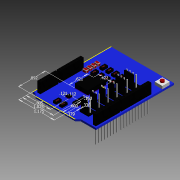
# Autodesk Inventor part: GBS-20132-EL2
Saved by Autodesk Inventor 2013 (Build 170138000, 138)
## iProperties
Created: 2013-09-06
Part Number: GBS-20132-EL2
Material: Generic
Document SubType Name: Modeling
Designer: HP_Administrator
Density: 1 g/cm^3
GlobalPropertyList: <PropertyList/>
Author: HP_Administrator
Autodesk Inventor part; units mm, degrees
(part 1 of 2)
ref_plane "YZ Plane" through (0, 0, 0) normal (1, 0, 0) x (0, 1, 0)
ref_plane "XZ Plane" through (0, 0, 0) normal (0, 1, 0) x (-1, 0, 0)
ref_plane "XY Plane" through (0, 0, 0) normal (0, 0, 1) x (1, 0, 0)
sketch "Sketch1" plane through (0, 0, 0) normal (0, 1, 0) x (-1, 0, 0)
  line L0 (26.67, -33.02) -> (-26.67, -33.02)
  line L1 (-26.67, -33.02) -> (-26.67, 33.02)
  line L2 (26.67, -33.02) -> (26.67, 33.02)
  line L3 (26.67, 33.02) -> (24.638, 33.02)
  line L4 (-26.67, 33.02) -> (-13.97, 33.02)
  line L5 (22.0345, 35.306) -> (-11.3665, 35.306)
  line L6 (24.638, 33.02) -> (22.0345, 35.306)
  line L7 (-11.3665, 35.306) -> (-13.97, 33.02)
  line L8 (26.67, -33.02) -> (-26.67, 33.02) construction
  line L9 (26.67, 33.02) -> (-26.67, -33.02) construction
  point P0 (0, 0)
  point P1 (0, 0)
  point P2 (0, 0)
  dimension "d0" = 53.34
  dimension "d1" = 66.04
  dimension "d2" = 66.04
  dimension "d3" = 2.032
  dimension "d4" = 12.7
  dimension "d5" = 2.286
  dimension "d6" = 33.401
  constraints: 20 end point, 2 midpoint, 2 parallel, 2 perpendicular, 1 coincident, 1 collinear, 1 equal length, 1 horizontal
  measures "d0" distance of L0.start L0.end
  measures "d1" distance of L0.end L1.end
  measures "d2" distance of L0.start L2.end
  measures "d3" distance of L2.end L3.end
  measures "d4" distance of L1.end L4.end
  measures "d5" distance between parallel lines of L4 L5
  measures "d6" distance of L5.start L5.end
extrude "PCB BD" add sketch "Sketch1" along normal blind 1.524
sketch "Sketch2" plane through (0, 1.524, 0) normal (0, 1, 0) x (1, 0, 0)
  line L0 (26.67, 33.02) -> (-26.67, 33.02) projected
  line L1 (-22.0345, -35.306) -> (11.3665, -35.306) projected
  line L2 (26.67, -33.02) -> (26.67, 33.02) projected
  line L3 (-4.8895, -32.766) -> (-2.2225, -32.766)
  line L4 (-2.2225, -32.766) -> (-2.2225, -28.1305)
  line L5 (-2.2225, -28.1305) -> (-4.8895, -28.1305)
  line L6 (-4.8895, -28.1305) -> (-4.8895, -32.766)
  line L7 (-7.1755, -32.766) -> (-9.8425, -32.766)
  line L8 (-9.8425, -32.766) -> (-9.8425, -28.1305)
  line L9 (-9.8425, -28.1305) -> (-7.1755, -28.1305)
  line L10 (-7.1755, -28.1305) -> (-7.1755, -32.766)
  line L11 (-0.127, 16.2179) -> (2.54, 16.2179)
  line L12 (2.54, 16.2179) -> (2.54, 11.5824)
  line L13 (2.54, 11.5824) -> (-0.127, 11.5824)
  line L14 (-0.127, 11.5824) -> (-0.127, 16.2179)
  line L15 (-2.413, 11.5824) -> (-5.08, 11.5824)
  line L16 (-5.08, 11.5824) -> (-5.08, 16.2179)
  line L17 (-5.08, 16.2179) -> (-2.413, 16.2179)
  line L18 (-2.413, 16.2179) -> (-2.413, 11.5824)
  line L19 (-7.366, 11.5824) -> (-10.033, 11.5824)
  line L20 (-10.033, 11.5824) -> (-10.033, 16.2179)
  line L21 (-10.033, 16.2179) -> (-7.366, 16.2179)
  line L22 (-7.366, 16.2179) -> (-7.366, 11.5824)
  line L23 (-12.319, 11.5824) -> (-14.986, 11.5824)
  line L24 (-14.986, 11.5824) -> (-14.986, 16.2179)
  line L25 (-14.986, 16.2179) -> (-12.319, 16.2179)
  line L26 (-12.319, 16.2179) -> (-12.319, 11.5824)
  line L27 (-14.986, 8.5344) -> (-12.319, 8.5344)
  line L28 (-12.319, 8.5344) -> (-12.319, 3.8989)
  line L29 (-12.319, 3.8989) -> (-14.986, 3.8989)
  line L30 (-14.986, 3.8989) -> (-14.986, 8.5344)
  line L31 (-10.033, 8.5344) -> (-7.366, 8.5344)
  line L32 (-7.366, 8.5344) -> (-7.366, 3.8989)
  line L33 (-7.366, 3.8989) -> (-10.033, 3.8989)
  line L34 (-10.033, 3.8989) -> (-10.033, 8.5344)
  line L35 (-5.08, 8.5344) -> (-2.413, 8.5344)
  line L36 (-2.413, 8.5344) -> (-2.413, 3.8989)
  line L37 (-2.413, 3.8989) -> (-5.08, 3.8989)
  line L38 (-5.08, 3.8989) -> (-5.08, 8.5344)
  line L39 (-0.127, 8.5344) -> (2.54, 8.5344)
  line L40 (2.54, 8.5344) -> (2.54, 3.8989)
  line L41 (2.54, 3.8989) -> (-0.127, 3.8989)
  line L42 (-0.127, 3.8989) -> (-0.127, 8.5344)
  point P0 (0, 0)
  dimension "d9" = 2.54
  dimension "d10" = 4.6355
  dimension "d11" = 2.667
  dimension "d13" = 28.8925
  dimension "d14" = 2.286
  dimension "d15" = 16.8021
  dimension "d16" = 24.13
  dimension "d17" = 2.286
  dimension "d18" = 2.286
  dimension "d19" = 2.286
  dimension "d20" = 3.048
  constraints: 80 end point, 20 parallel, 18 equal length, 11 collinear, 10 horizontal, 10 perpendicular
  measures "d9" distance between parallel lines of L1 L3
  measures "d10" distance of L3.end L4.end
  measures "d11" distance of L4.end L5.end
  measures "d13" distance between parallel lines of L2 L4
  measures "d14" distance between parallel lines of L10 L6
  measures "d15" distance between parallel lines of L0 L11
  measures "d16" distance between parallel lines of L2 L12
  measures "d17" distance between parallel lines of L18 L14
  measures "d18" distance between parallel lines of L22 L16
  measures "d19" distance between parallel lines of L26 L20
  measures "d20" distance between parallel lines of L27 L23
extrude "SK14 GP" add sketch "Sketch2" along normal blind 1.778
sketch "Sketch3" plane through (0, 3.302, 0) normal (0, 1, 0) x (1, 0, 0)
  line L0 (-2.2225, -32.766) -> (-2.2225, -28.1305) projected
  line L1 (-14.986, 11.5824) -> (-12.319, 11.5824) projected
  line L2 (-12.319, 11.5824) -> (-12.319, 16.2179) projected
  line L3 (-12.319, 16.2179) -> (-14.986, 16.2179) projected
  line L4 (-14.986, 16.2179) -> (-14.986, 11.5824) projected
  line L5 (-10.033, 11.5824) -> (-7.366, 11.5824) projected
  line L6 (-7.366, 11.5824) -> (-7.366, 16.2179) projected
  line L7 (-7.366, 16.2179) -> (-10.033, 16.2179) projected
  line L8 (-10.033, 16.2179) -> (-10.033, 11.5824) projected
  line L9 (-5.08, 11.5824) -> (-2.413, 11.5824) projected
  line L10 (-2.413, 11.5824) -> (-2.413, 16.2179) projected
  line L11 (-2.413, 16.2179) -> (-5.08, 16.2179) projected
  line L12 (-5.08, 16.2179) -> (-5.08, 11.5824) projected
  line L13 (2.54, 16.2179) -> (-0.127, 16.2179) projected
  line L14 (-0.127, 16.2179) -> (-0.127, 11.5824) projected
  line L15 (-0.127, 11.5824) -> (2.54, 11.5824) projected
  line L16 (2.54, 11.5824) -> (2.54, 16.2179) projected
  line L17 (2.54, 8.5344) -> (-0.127, 8.5344) projected
  line L18 (-0.127, 8.5344) -> (-0.127, 3.8989) projected
  line L19 (-0.127, 3.8989) -> (2.54, 3.8989) projected
  line L20 (2.54, 3.8989) -> (2.54, 8.5344) projected
  line L21 (-2.413, 8.5344) -> (-5.08, 8.5344) projected
  line L22 (-5.08, 8.5344) -> (-5.08, 3.8989) projected
  line L23 (-5.08, 3.8989) -> (-2.413, 3.8989) projected
  line L24 (-2.413, 3.8989) -> (-2.413, 8.5344) projected
  line L25 (-7.366, 8.5344) -> (-10.033, 8.5344) projected
  line L26 (-10.033, 8.5344) -> (-10.033, 3.8989) projected
  line L27 (-10.033, 3.8989) -> (-7.366, 3.8989) projected
  line L28 (-7.366, 3.8989) -> (-7.366, 8.5344) projected
  line L29 (-12.319, 8.5344) -> (-14.986, 8.5344) projected
  line L30 (-14.986, 8.5344) -> (-14.986, 3.8989) projected
  line L31 (-14.986, 3.8989) -> (-12.319, 3.8989) projected
  line L32 (-12.319, 3.8989) -> (-12.319, 8.5344) projected
  line L33 (-9.8425, -32.766) -> (-7.1755, -32.766) projected
  line L34 (-9.8425, -32.766) -> (-7.1755, -32.766) projected
  line L35 (-7.1755, -32.766) -> (-7.1755, -28.1305) projected
  line L36 (-7.1755, -28.1305) -> (-9.8425, -28.1305) projected
  line L37 (-9.8425, -28.1305) -> (-9.8425, -32.766) projected
  line L38 (-7.6327, -29.7815) -> (-7.6327, -32.766) construction
  line L39 (-7.6327, -32.766) -> (-9.8425, -32.766) construction
  line L40 (-9.8425, -32.766) -> (-9.8425, -29.7815) construction
  line L41 (-9.8425, -29.7815) -> (-7.6327, -29.7815) construction
  line L42 (-2.6797, -29.7815) -> (-2.6797, -32.766) construction
  line L43 (-2.6797, -32.766) -> (-4.8895, -32.766) construction
  line L44 (-4.8895, -32.766) -> (-4.8895, -29.7815) construction
  line L45 (-4.8895, -29.7815) -> (-2.6797, -29.7815) construction
  line L46 (2.0828, 14.5669) -> (2.0828, 11.5824) construction
  line L47 (2.0828, 11.5824) -> (-0.127, 11.5824) construction
  line L48 (-0.127, 11.5824) -> (-0.127, 14.5669) construction
  line L49 (-0.127, 14.5669) -> (2.0828, 14.5669) construction
  line L50 (-12.9587, 6.8834) -> (-12.9587, 3.8989) construction
  line L51 (-12.9587, 3.8989) -> (-14.986, 3.8989) construction
  line L52 (-14.986, 3.8989) -> (-14.986, 6.8834) construction
  line L53 (-14.986, 6.8834) -> (-12.9587, 6.8834) construction
  line L54 (-7.8232, 6.8834) -> (-7.8232, 3.8989) construction
  line L55 (-7.8232, 3.8989) -> (-10.033, 3.8989) construction
  line L56 (-10.033, 3.8989) -> (-10.033, 6.8834) construction
  line L57 (-10.033, 6.8834) -> (-7.8232, 6.8834) construction
  line L58 (-12.9587, 14.5669) -> (-12.9587, 11.5824) construction
  line L59 (-12.9587, 11.5824) -> (-14.986, 11.5824) construction
  line L60 (-14.986, 11.5824) -> (-14.986, 14.5669) construction
  line L61 (-14.986, 14.5669) -> (-12.9587, 14.5669) construction
  line L62 (-7.8232, 14.5669) -> (-7.8232, 11.5824) construction
  line L63 (-7.8232, 11.5824) -> (-10.033, 11.5824) construction
  line L64 (-10.033, 11.5824) -> (-10.033, 14.5669) construction
  line L65 (-10.033, 14.5669) -> (-7.8232, 14.5669) construction
  line L66 (-2.8702, 14.5669) -> (-2.8702, 11.5824) construction
  line L67 (-2.8702, 11.5824) -> (-5.08, 11.5824) construction
  line L68 (-5.08, 11.5824) -> (-5.08, 14.5669) construction
  line L69 (-5.08, 14.5669) -> (-2.8702, 14.5669) construction
  line L70 (-5.08, 6.8834) -> (-2.8702, 6.8834) construction
  line L71 (-2.8702, 6.8834) -> (-2.8702, 3.8989) construction
  line L72 (-2.8702, 3.8989) -> (-5.08, 3.8989) construction
  line L73 (-5.08, 3.8989) -> (-5.08, 6.8834) construction
  line L74 (-0.127, 6.8834) -> (2.0828, 6.8834) construction
  line L75 (2.0828, 6.8834) -> (2.0828, 3.8989) construction
  line L76 (2.0828, 3.8989) -> (-0.127, 3.8989) construction
  line L77 (-0.127, 3.8989) -> (-0.127, 6.8834) construction
  spline S0 degree 2 poles (-8.4482, -30.0808) (-8.4482, -29.9953) (-8.4124, -29.8753) (-8.3869, -29.8223) knots 0 0 0 1 2 2 2
  line L78 (-8.3869, -29.8223) -> (-8.2555, -29.8223)
  line L79 (-8.2555, -29.8223) -> (-8.2555, -29.83)
  spline S1 degree 2 poles (-8.2555, -29.83) (-8.304, -29.8817) (-8.3576, -30.0125) (-8.3576, -30.0731) knots 0 0 0 1 2 2 2
  spline S2 degree 2 poles (-8.3576, -30.0731) (-8.3576, -30.1599) (-8.2855, -30.2486) (-8.2261, -30.2486) knots 0 0 0 1 2 2 2
  spline S3 degree 2 poles (-8.2261, -30.2486) (-8.1789, -30.2486) (-8.1202, -30.202) (-8.1055, -30.1516) knots 0 0 0 1 2 2 2
  spline S4 degree 2 poles (-8.1055, -30.1516) (-8.0953, -30.1152) (-8.0813, -30.0546) (-8.0698, -30.0093) knots 0 0 0 1 2 2 2
  spline S5 degree 2 poles (-8.0698, -30.0093) (-8.0589, -29.9685) (-8.0264, -29.904) (-8.0002, -29.8791) knots 0 0 0 1 2 2 2
  spline S6 degree 2 poles (-8.0002, -29.8791) (-7.9741, -29.8549) (-7.9039, -29.8281) (-7.8579, -29.8281) knots 0 0 0 1 2 2 2
  spline S7 degree 2 poles (-7.8579, -29.8281) (-7.7622, -29.8281) (-7.6327, -29.9774) (-7.6327, -30.0929) knots 0 0 0 1 2 2 2
  spline S8 degree 2 poles (-7.6327, -30.0929) (-7.6327, -30.1592) (-7.6589, -30.2767) (-7.6837, -30.3271) knots 0 0 0 1 2 2 2
  line L80 (-7.6837, -30.3271) -> (-7.8088, -30.3271)
  line L81 (-7.8088, -30.3271) -> (-7.8088, -30.3194)
  spline S9 degree 2 poles (-7.8088, -30.3194) (-7.7744, -30.2818) (-7.7233, -30.1644) (-7.7233, -30.0999) knots 0 0 0 1 2 2 2
  spline S10 degree 2 poles (-7.7233, -30.0999) (-7.7233, -30.0272) (-7.7916, -29.9372) (-7.8471, -29.9372) knots 0 0 0 1 2 2 2
  spline S11 degree 2 poles (-7.8471, -29.9372) (-7.8969, -29.9372) (-7.9562, -29.9902) (-7.9696, -30.0399) knots 0 0 0 1 2 2 2
  spline S12 degree 2 poles (-7.9696, -30.0399) (-7.9785, -30.0731) (-8.0015, -30.1695) (-8.0111, -30.2014) knots 0 0 0 1 2 2 2
  spline S13 degree 2 poles (-8.0111, -30.2014) (-8.036, -30.2824) (-8.1362, -30.3577) (-8.2095, -30.3577) knots 0 0 0 1 2 2 2
  spline S14 degree 2 poles (-8.2095, -30.3577) (-8.2561, -30.3577) (-8.3454, -30.32) (-8.3767, -30.2862) knots 0 0 0 1 2 2 2
  spline S15 degree 2 poles (-8.3767, -30.2862) (-8.4112, -30.2486) (-8.4482, -30.1529) (-8.4482, -30.0808) knots 0 0 0 1 2 2 2
  line L82 (-8.4341, -31.0385) -> (-8.4341, -30.9026)
  line L83 (-8.4341, -30.9026) -> (-8.0679, -30.6148)
  line L84 (-8.0679, -30.6148) -> (-8.1196, -30.5689)
  line L85 (-8.1196, -30.5689) -> (-8.4341, -30.5689)
  line L86 (-8.4341, -30.5689) -> (-8.4341, -30.4643)
  line L87 (-8.4341, -30.4643) -> (-7.6467, -30.4643)
  line L88 (-7.6467, -30.4643) -> (-7.6467, -30.5689)
  line L89 (-7.6467, -30.5689) -> (-8.0085, -30.5689)
  line L90 (-8.0085, -30.5689) -> (-7.6467, -30.8918)
  line L91 (-7.6467, -30.8918) -> (-7.6467, -31.0194)
  line L92 (-7.6467, -31.0194) -> (-7.9983, -30.6933)
  line L93 (-7.9983, -30.6933) -> (-8.4341, -31.0385)
  line L94 (-8.4341, -31.5248) -> (-8.4341, -31.1406)
  line L95 (-8.4341, -31.1406) -> (-8.3537, -31.1406)
  line L96 (-8.3537, -31.1406) -> (-8.3537, -31.2836)
  line L97 (-8.3537, -31.2836) -> (-7.826, -31.2836)
  line L98 (-7.826, -31.2836) -> (-7.826, -31.1406)
  line L99 (-7.826, -31.1406) -> (-7.7539, -31.1406)
  spline S16 degree 2 poles (-7.7539, -31.1406) (-7.7539, -31.2217) (-7.708, -31.2982) (-7.6442, -31.3033) knots 0 0 0 1 2 2 2
  line L100 (-7.6442, -31.3033) -> (-7.6442, -31.385)
  line L101 (-7.6442, -31.385) -> (-8.3537, -31.385)
  line L102 (-8.3537, -31.385) -> (-8.3537, -31.5248)
  line L103 (-8.3537, -31.5248) -> (-8.4341, -31.5248)
  line L104 (-8.1636, -32.1762) -> (-8.1636, -32.0824)
  line L105 (-8.1636, -32.0824) -> (-8.4341, -32.0824)
  line L106 (-8.4341, -32.0824) -> (-8.4341, -31.981)
  line L107 (-8.4341, -31.981) -> (-8.1636, -31.981)
  line L108 (-8.1636, -31.981) -> (-8.1636, -31.6332)
  line L109 (-8.1636, -31.6332) -> (-8.0526, -31.6332)
  line L110 (-8.0526, -31.6332) -> (-7.6467, -31.9855)
  line L111 (-7.6467, -31.9855) -> (-7.6467, -32.0824)
  line L112 (-7.6467, -32.0824) -> (-8.0787, -32.0824)
  line L113 (-8.0787, -32.0824) -> (-8.0787, -32.1762)
  line L114 (-8.0787, -32.1762) -> (-8.1636, -32.1762)
  line L115 (-8.0787, -31.981) -> (-7.7712, -31.981)
  line L116 (-7.7712, -31.981) -> (-8.0787, -31.7162)
  line L117 (-8.0787, -31.7162) -> (-8.0787, -31.981)
  spline S17 degree 2 poles (-3.4952, -30.0808) (-3.4952, -29.9953) (-3.4594, -29.8753) (-3.4339, -29.8223) knots 0 0 0 1 2 2 2
  line L118 (-3.4339, -29.8223) -> (-3.3025, -29.8223)
  line L119 (-3.3025, -29.8223) -> (-3.3025, -29.83)
  spline S18 degree 2 poles (-3.3025, -29.83) (-3.351, -29.8817) (-3.4046, -30.0125) (-3.4046, -30.0731) knots 0 0 0 1 2 2 2
  spline S19 degree 2 poles (-3.4046, -30.0731) (-3.4046, -30.1599) (-3.3325, -30.2486) (-3.2731, -30.2486) knots 0 0 0 1 2 2 2
  spline S20 degree 2 poles (-3.2731, -30.2486) (-3.2259, -30.2486) (-3.1672, -30.202) (-3.1525, -30.1516) knots 0 0 0 1 2 2 2
  spline S21 degree 2 poles (-3.1525, -30.1516) (-3.1423, -30.1152) (-3.1283, -30.0546) (-3.1168, -30.0093) knots 0 0 0 1 2 2 2
  spline S22 degree 2 poles (-3.1168, -30.0093) (-3.1059, -29.9685) (-3.0734, -29.904) (-3.0472, -29.8791) knots 0 0 0 1 2 2 2
  spline S23 degree 2 poles (-3.0472, -29.8791) (-3.0211, -29.8549) (-2.9509, -29.8281) (-2.9049, -29.8281) knots 0 0 0 1 2 2 2
  spline S24 degree 2 poles (-2.9049, -29.8281) (-2.8092, -29.8281) (-2.6797, -29.9774) (-2.6797, -30.0929) knots 0 0 0 1 2 2 2
  spline S25 degree 2 poles (-2.6797, -30.0929) (-2.6797, -30.1592) (-2.7059, -30.2767) (-2.7307, -30.3271) knots 0 0 0 1 2 2 2
  line L120 (-2.7307, -30.3271) -> (-2.8558, -30.3271)
  line L121 (-2.8558, -30.3271) -> (-2.8558, -30.3194)
  spline S26 degree 2 poles (-2.8558, -30.3194) (-2.8214, -30.2818) (-2.7703, -30.1644) (-2.7703, -30.0999) knots 0 0 0 1 2 2 2
  spline S27 degree 2 poles (-2.7703, -30.0999) (-2.7703, -30.0272) (-2.8386, -29.9372) (-2.8941, -29.9372) knots 0 0 0 1 2 2 2
  spline S28 degree 2 poles (-2.8941, -29.9372) (-2.9439, -29.9372) (-3.0032, -29.9902) (-3.0166, -30.0399) knots 0 0 0 1 2 2 2
  spline S29 degree 2 poles (-3.0166, -30.0399) (-3.0255, -30.0731) (-3.0485, -30.1695) (-3.0581, -30.2014) knots 0 0 0 1 2 2 2
  spline S30 degree 2 poles (-3.0581, -30.2014) (-3.083, -30.2824) (-3.1832, -30.3577) (-3.2565, -30.3577) knots 0 0 0 1 2 2 2
  spline S31 degree 2 poles (-3.2565, -30.3577) (-3.3031, -30.3577) (-3.3924, -30.32) (-3.4237, -30.2862) knots 0 0 0 1 2 2 2
  spline S32 degree 2 poles (-3.4237, -30.2862) (-3.4582, -30.2486) (-3.4952, -30.1529) (-3.4952, -30.0808) knots 0 0 0 1 2 2 2
  line L122 (-3.4811, -31.0385) -> (-3.4811, -30.9026)
  line L123 (-3.4811, -30.9026) -> (-3.1149, -30.6148)
  line L124 (-3.1149, -30.6148) -> (-3.1666, -30.5689)
  line L125 (-3.1666, -30.5689) -> (-3.4811, -30.5689)
  line L126 (-3.4811, -30.5689) -> (-3.4811, -30.4643)
  line L127 (-3.4811, -30.4643) -> (-2.6937, -30.4643)
  line L128 (-2.6937, -30.4643) -> (-2.6937, -30.5689)
  line L129 (-2.6937, -30.5689) -> (-3.0555, -30.5689)
  line L130 (-3.0555, -30.5689) -> (-2.6937, -30.8918)
  line L131 (-2.6937, -30.8918) -> (-2.6937, -31.0194)
  line L132 (-2.6937, -31.0194) -> (-3.0453, -30.6933)
  line L133 (-3.0453, -30.6933) -> (-3.4811, -31.0385)
  line L134 (-3.4811, -31.5248) -> (-3.4811, -31.1406)
  line L135 (-3.4811, -31.1406) -> (-3.4007, -31.1406)
  line L136 (-3.4007, -31.1406) -> (-3.4007, -31.2836)
  line L137 (-3.4007, -31.2836) -> (-2.873, -31.2836)
  line L138 (-2.873, -31.2836) -> (-2.873, -31.1406)
  line L139 (-2.873, -31.1406) -> (-2.8009, -31.1406)
  spline S33 degree 2 poles (-2.8009, -31.1406) (-2.8009, -31.2217) (-2.755, -31.2982) (-2.6912, -31.3033) knots 0 0 0 1 2 2 2
  line L140 (-2.6912, -31.3033) -> (-2.6912, -31.385)
  line L141 (-2.6912, -31.385) -> (-3.4007, -31.385)
  line L142 (-3.4007, -31.385) -> (-3.4007, -31.5248)
  line L143 (-3.4007, -31.5248) -> (-3.4811, -31.5248)
  line L144 (-3.2106, -32.1762) -> (-3.2106, -32.0824)
  line L145 (-3.2106, -32.0824) -> (-3.4811, -32.0824)
  line L146 (-3.4811, -32.0824) -> (-3.4811, -31.981)
  line L147 (-3.4811, -31.981) -> (-3.2106, -31.981)
  line L148 (-3.2106, -31.981) -> (-3.2106, -31.6332)
  line L149 (-3.2106, -31.6332) -> (-3.0996, -31.6332)
  line L150 (-3.0996, -31.6332) -> (-2.6937, -31.9855)
  line L151 (-2.6937, -31.9855) -> (-2.6937, -32.0824)
  line L152 (-2.6937, -32.0824) -> (-3.1257, -32.0824)
  line L153 (-3.1257, -32.0824) -> (-3.1257, -32.1762)
  line L154 (-3.1257, -32.1762) -> (-3.2106, -32.1762)
  line L155 (-3.1257, -31.981) -> (-2.8182, -31.981)
  line L156 (-2.8182, -31.981) -> (-3.1257, -31.7162)
  line L157 (-3.1257, -31.7162) -> (-3.1257, -31.981)
  spline S34 degree 2 poles (-13.7742, 6.5841) (-13.7742, 6.6696) (-13.7384, 6.7896) (-13.7129, 6.8426) knots 0 0 0 1 2 2 2
  line L158 (-13.7129, 6.8426) -> (-13.5815, 6.8426)
  line L159 (-13.5815, 6.8426) -> (-13.5815, 6.8349)
  spline S35 degree 2 poles (-13.5815, 6.8349) (-13.63, 6.7832) (-13.6836, 6.6524) (-13.6836, 6.5918) knots 0 0 0 1 2 2 2
  spline S36 degree 2 poles (-13.6836, 6.5918) (-13.6836, 6.505) (-13.6114, 6.4163) (-13.5521, 6.4163) knots 0 0 0 1 2 2 2
  spline S37 degree 2 poles (-13.5521, 6.4163) (-13.5049, 6.4163) (-13.4462, 6.4629) (-13.4315, 6.5133) knots 0 0 0 1 2 2 2
  spline S38 degree 2 poles (-13.4315, 6.5133) (-13.4213, 6.5497) (-13.4073, 6.6103) (-13.3958, 6.6556) knots 0 0 0 1 2 2 2
  spline S39 degree 2 poles (-13.3958, 6.6556) (-13.3849, 6.6964) (-13.3524, 6.7609) (-13.3262, 6.7858) knots 0 0 0 1 2 2 2
  spline S40 degree 2 poles (-13.3262, 6.7858) (-13.3001, 6.81) (-13.2299, 6.8368) (-13.1839, 6.8368) knots 0 0 0 1 2 2 2
  spline S41 degree 2 poles (-13.1839, 6.8368) (-13.0882, 6.8368) (-12.9587, 6.6875) (-12.9587, 6.572) knots 0 0 0 1 2 2 2
  spline S42 degree 2 poles (-12.9587, 6.572) (-12.9587, 6.5057) (-12.9848, 6.3882) (-13.0097, 6.3378) knots 0 0 0 1 2 2 2
  line L160 (-13.0097, 6.3378) -> (-13.1348, 6.3378)
  line L161 (-13.1348, 6.3378) -> (-13.1348, 6.3455)
  spline S43 degree 2 poles (-13.1348, 6.3455) (-13.1003, 6.3831) (-13.0493, 6.5005) (-13.0493, 6.565) knots 0 0 0 1 2 2 2
  spline S44 degree 2 poles (-13.0493, 6.565) (-13.0493, 6.6377) (-13.1176, 6.7277) (-13.1731, 6.7277) knots 0 0 0 1 2 2 2
  spline S45 degree 2 poles (-13.1731, 6.7277) (-13.2229, 6.7277) (-13.2822, 6.6747) (-13.2956, 6.625) knots 0 0 0 1 2 2 2
  spline S46 degree 2 poles (-13.2956, 6.625) (-13.3045, 6.5918) (-13.3275, 6.4954) (-13.3371, 6.4635) knots 0 0 0 1 2 2 2
  spline S47 degree 2 poles (-13.3371, 6.4635) (-13.362, 6.3825) (-13.4621, 6.3072) (-13.5355, 6.3072) knots 0 0 0 1 2 2 2
  spline S48 degree 2 poles (-13.5355, 6.3072) (-13.5821, 6.3072) (-13.6714, 6.3449) (-13.7027, 6.3787) knots 0 0 0 1 2 2 2
  spline S49 degree 2 poles (-13.7027, 6.3787) (-13.7372, 6.4163) (-13.7742, 6.512) (-13.7742, 6.5841) knots 0 0 0 1 2 2 2
  line L162 (-13.7601, 5.6264) -> (-13.7601, 5.7623)
  line L163 (-13.7601, 5.7623) -> (-13.3939, 6.0501)
  line L164 (-13.3939, 6.0501) -> (-13.4455, 6.096)
  line L165 (-13.4455, 6.096) -> (-13.7601, 6.096)
  line L166 (-13.7601, 6.096) -> (-13.7601, 6.2006)
  line L167 (-13.7601, 6.2006) -> (-12.9727, 6.2006)
  line L168 (-12.9727, 6.2006) -> (-12.9727, 6.096)
  line L169 (-12.9727, 6.096) -> (-13.3345, 6.096)
  line L170 (-13.3345, 6.096) -> (-12.9727, 5.7731)
  line L171 (-12.9727, 5.7731) -> (-12.9727, 5.6455)
  line L172 (-12.9727, 5.6455) -> (-13.3243, 5.9716)
  line L173 (-13.3243, 5.9716) -> (-13.7601, 5.6264)
  line L174 (-13.7601, 5.1401) -> (-13.7601, 5.5243)
  line L175 (-13.7601, 5.5243) -> (-13.6797, 5.5243)
  line L176 (-13.6797, 5.5243) -> (-13.6797, 5.3813)
  line L177 (-13.6797, 5.3813) -> (-13.152, 5.3813)
  line L178 (-13.152, 5.3813) -> (-13.152, 5.5243)
  line L179 (-13.152, 5.5243) -> (-13.0799, 5.5243)
  spline S50 degree 2 poles (-13.0799, 5.5243) (-13.0799, 5.4432) (-13.034, 5.3667) (-12.9702, 5.3616) knots 0 0 0 1 2 2 2
  line L180 (-12.9702, 5.3616) -> (-12.9702, 5.2799)
  line L181 (-12.9702, 5.2799) -> (-13.6797, 5.2799)
  line L182 (-13.6797, 5.2799) -> (-13.6797, 5.1401)
  line L183 (-13.6797, 5.1401) -> (-13.7601, 5.1401)
  line L184 (-13.4896, 4.4887) -> (-13.4896, 4.5825)
  line L185 (-13.4896, 4.5825) -> (-13.7601, 4.5825)
  line L186 (-13.7601, 4.5825) -> (-13.7601, 4.6839)
  line L187 (-13.7601, 4.6839) -> (-13.4896, 4.6839)
  line L188 (-13.4896, 4.6839) -> (-13.4896, 5.0317)
  line L189 (-13.4896, 5.0317) -> (-13.3785, 5.0317)
  line L190 (-13.3785, 5.0317) -> (-12.9727, 4.6794)
  line L191 (-12.9727, 4.6794) -> (-12.9727, 4.5825)
  line L192 (-12.9727, 4.5825) -> (-13.4047, 4.5825)
  line L193 (-13.4047, 4.5825) -> (-13.4047, 4.4887)
  line L194 (-13.4047, 4.4887) -> (-13.4896, 4.4887)
  line L195 (-13.4047, 4.6839) -> (-13.0971, 4.6839)
  line L196 (-13.0971, 4.6839) -> (-13.4047, 4.9487)
  line L197 (-13.4047, 4.9487) -> (-13.4047, 4.6839)
  spline S51 degree 2 poles (-13.7742, 14.2676) (-13.7742, 14.3531) (-13.7384, 14.4731) (-13.7129, 14.5261) knots 0 0 0 1 2 2 2
  line L198 (-13.7129, 14.5261) -> (-13.5815, 14.5261)
  line L199 (-13.5815, 14.5261) -> (-13.5815, 14.5184)
  spline S52 degree 2 poles (-13.5815, 14.5184) (-13.63, 14.4667) (-13.6836, 14.3359) (-13.6836, 14.2753) knots 0 0 0 1 2 2 2
  spline S53 degree 2 poles (-13.6836, 14.2753) (-13.6836, 14.1885) (-13.6114, 14.0998) (-13.5521, 14.0998) knots 0 0 0 1 2 2 2
  spline S54 degree 2 poles (-13.5521, 14.0998) (-13.5049, 14.0998) (-13.4462, 14.1464) (-13.4315, 14.1968) knots 0 0 0 1 2 2 2
  spline S55 degree 2 poles (-13.4315, 14.1968) (-13.4213, 14.2332) (-13.4073, 14.2938) (-13.3958, 14.3391) knots 0 0 0 1 2 2 2
  spline S56 degree 2 poles (-13.3958, 14.3391) (-13.3849, 14.3799) (-13.3524, 14.4444) (-13.3262, 14.4693) knots 0 0 0 1 2 2 2
  spline S57 degree 2 poles (-13.3262, 14.4693) (-13.3001, 14.4935) (-13.2299, 14.5203) (-13.1839, 14.5203) knots 0 0 0 1 2 2 2
  spline S58 degree 2 poles (-13.1839, 14.5203) (-13.0882, 14.5203) (-12.9587, 14.371) (-12.9587, 14.2555) knots 0 0 0 1 2 2 2
  spline S59 degree 2 poles (-12.9587, 14.2555) (-12.9587, 14.1892) (-12.9848, 14.0717) (-13.0097, 14.0213) knots 0 0 0 1 2 2 2
  line L200 (-13.0097, 14.0213) -> (-13.1348, 14.0213)
  line L201 (-13.1348, 14.0213) -> (-13.1348, 14.029)
  spline S60 degree 2 poles (-13.1348, 14.029) (-13.1003, 14.0666) (-13.0493, 14.184) (-13.0493, 14.2485) knots 0 0 0 1 2 2 2
  spline S61 degree 2 poles (-13.0493, 14.2485) (-13.0493, 14.3212) (-13.1176, 14.4112) (-13.1731, 14.4112) knots 0 0 0 1 2 2 2
  spline S62 degree 2 poles (-13.1731, 14.4112) (-13.2229, 14.4112) (-13.2822, 14.3582) (-13.2956, 14.3085) knots 0 0 0 1 2 2 2
  spline S63 degree 2 poles (-13.2956, 14.3085) (-13.3045, 14.2753) (-13.3275, 14.1789) (-13.3371, 14.147) knots 0 0 0 1 2 2 2
  spline S64 degree 2 poles (-13.3371, 14.147) (-13.362, 14.066) (-13.4621, 13.9907) (-13.5355, 13.9907) knots 0 0 0 1 2 2 2
  spline S65 degree 2 poles (-13.5355, 13.9907) (-13.5821, 13.9907) (-13.6714, 14.0284) (-13.7027, 14.0622) knots 0 0 0 1 2 2 2
  spline S66 degree 2 poles (-13.7027, 14.0622) (-13.7372, 14.0998) (-13.7742, 14.1955) (-13.7742, 14.2676) knots 0 0 0 1 2 2 2
  line L202 (-13.7601, 13.3099) -> (-13.7601, 13.4458)
  line L203 (-13.7601, 13.4458) -> (-13.3939, 13.7336)
  line L204 (-13.3939, 13.7336) -> (-13.4455, 13.7795)
  line L205 (-13.4455, 13.7795) -> (-13.7601, 13.7795)
  line L206 (-13.7601, 13.7795) -> (-13.7601, 13.8841)
  line L207 (-13.7601, 13.8841) -> (-12.9727, 13.8841)
  line L208 (-12.9727, 13.8841) -> (-12.9727, 13.7795)
  line L209 (-12.9727, 13.7795) -> (-13.3345, 13.7795)
  line L210 (-13.3345, 13.7795) -> (-12.9727, 13.4566)
  line L211 (-12.9727, 13.4566) -> (-12.9727, 13.329)
  line L212 (-12.9727, 13.329) -> (-13.3243, 13.6551)
  line L213 (-13.3243, 13.6551) -> (-13.7601, 13.3099)
  line L214 (-13.7601, 12.8236) -> (-13.7601, 13.2078)
  line L215 (-13.7601, 13.2078) -> (-13.6797, 13.2078)
  line L216 (-13.6797, 13.2078) -> (-13.6797, 13.0648)
  line L217 (-13.6797, 13.0648) -> (-13.152, 13.0648)
  line L218 (-13.152, 13.0648) -> (-13.152, 13.2078)
  line L219 (-13.152, 13.2078) -> (-13.0799, 13.2078)
  spline S67 degree 2 poles (-13.0799, 13.2078) (-13.0799, 13.1267) (-13.034, 13.0502) (-12.9702, 13.0451) knots 0 0 0 1 2 2 2
  line L220 (-12.9702, 13.0451) -> (-12.9702, 12.9634)
  line L221 (-12.9702, 12.9634) -> (-13.6797, 12.9634)
  line L222 (-13.6797, 12.9634) -> (-13.6797, 12.8236)
  line L223 (-13.6797, 12.8236) -> (-13.7601, 12.8236)
  line L224 (-13.4896, 12.1722) -> (-13.4896, 12.266)
  line L225 (-13.4896, 12.266) -> (-13.7601, 12.266)
  line L226 (-13.7601, 12.266) -> (-13.7601, 12.3674)
  line L227 (-13.7601, 12.3674) -> (-13.4896, 12.3674)
  line L228 (-13.4896, 12.3674) -> (-13.4896, 12.7152)
  line L229 (-13.4896, 12.7152) -> (-13.3785, 12.7152)
  line L230 (-13.3785, 12.7152) -> (-12.9727, 12.3629)
  line L231 (-12.9727, 12.3629) -> (-12.9727, 12.266)
  line L232 (-12.9727, 12.266) -> (-13.4047, 12.266)
  line L233 (-13.4047, 12.266) -> (-13.4047, 12.1722)
  line L234 (-13.4047, 12.1722) -> (-13.4896, 12.1722)
  line L235 (-13.4047, 12.3674) -> (-13.0971, 12.3674)
  line L236 (-13.0971, 12.3674) -> (-13.4047, 12.6322)
  line L237 (-13.4047, 12.6322) -> (-13.4047, 12.3674)
  spline S68 degree 2 poles (-8.6387, 14.2676) (-8.6387, 14.3531) (-8.6029, 14.4731) (-8.5774, 14.5261) knots 0 0 0 1 2 2 2
  line L238 (-8.5774, 14.5261) -> (-8.446, 14.5261)
  line L239 (-8.446, 14.5261) -> (-8.446, 14.5184)
  spline S69 degree 2 poles (-8.446, 14.5184) (-8.4945, 14.4667) (-8.5481, 14.3359) (-8.5481, 14.2753) knots 0 0 0 1 2 2 2
  spline S70 degree 2 poles (-8.5481, 14.2753) (-8.5481, 14.1885) (-8.476, 14.0998) (-8.4166, 14.0998) knots 0 0 0 1 2 2 2
  spline S71 degree 2 poles (-8.4166, 14.0998) (-8.3694, 14.0998) (-8.3107, 14.1464) (-8.296, 14.1968) knots 0 0 0 1 2 2 2
  spline S72 degree 2 poles (-8.296, 14.1968) (-8.2858, 14.2332) (-8.2718, 14.2938) (-8.2603, 14.3391) knots 0 0 0 1 2 2 2
  spline S73 degree 2 poles (-8.2603, 14.3391) (-8.2494, 14.3799) (-8.2169, 14.4444) (-8.1907, 14.4693) knots 0 0 0 1 2 2 2
  spline S74 degree 2 poles (-8.1907, 14.4693) (-8.1646, 14.4935) (-8.0944, 14.5203) (-8.0484, 14.5203) knots 0 0 0 1 2 2 2
  spline S75 degree 2 poles (-8.0484, 14.5203) (-7.9527, 14.5203) (-7.8232, 14.371) (-7.8232, 14.2555) knots 0 0 0 1 2 2 2
  spline S76 degree 2 poles (-7.8232, 14.2555) (-7.8232, 14.1892) (-7.8494, 14.0717) (-7.8742, 14.0213) knots 0 0 0 1 2 2 2
  line L240 (-7.8742, 14.0213) -> (-7.9993, 14.0213)
  line L241 (-7.9993, 14.0213) -> (-7.9993, 14.029)
  spline S77 degree 2 poles (-7.9993, 14.029) (-7.9649, 14.0666) (-7.9138, 14.184) (-7.9138, 14.2485) knots 0 0 0 1 2 2 2
  spline S78 degree 2 poles (-7.9138, 14.2485) (-7.9138, 14.3212) (-7.9821, 14.4112) (-8.0376, 14.4112) knots 0 0 0 1 2 2 2
  spline S79 degree 2 poles (-8.0376, 14.4112) (-8.0874, 14.4112) (-8.1467, 14.3582) (-8.1601, 14.3085) knots 0 0 0 1 2 2 2
  spline S80 degree 2 poles (-8.1601, 14.3085) (-8.169, 14.2753) (-8.192, 14.1789) (-8.2016, 14.147) knots 0 0 0 1 2 2 2
  spline S81 degree 2 poles (-8.2016, 14.147) (-8.2265, 14.066) (-8.3267, 13.9907) (-8.4, 13.9907) knots 0 0 0 1 2 2 2
  spline S82 degree 2 poles (-8.4, 13.9907) (-8.4466, 13.9907) (-8.5359, 14.0284) (-8.5672, 14.0622) knots 0 0 0 1 2 2 2
  spline S83 degree 2 poles (-8.5672, 14.0622) (-8.6017, 14.0998) (-8.6387, 14.1955) (-8.6387, 14.2676) knots 0 0 0 1 2 2 2
  line L242 (-8.6246, 13.3099) -> (-8.6246, 13.4458)
  line L243 (-8.6246, 13.4458) -> (-8.2584, 13.7336)
  line L244 (-8.2584, 13.7336) -> (-8.3101, 13.7795)
  line L245 (-8.3101, 13.7795) -> (-8.6246, 13.7795)
  line L246 (-8.6246, 13.7795) -> (-8.6246, 13.8841)
  line L247 (-8.6246, 13.8841) -> (-7.8372, 13.8841)
  line L248 (-7.8372, 13.8841) -> (-7.8372, 13.7795)
  line L249 (-7.8372, 13.7795) -> (-8.199, 13.7795)
  line L250 (-8.199, 13.7795) -> (-7.8372, 13.4566)
  line L251 (-7.8372, 13.4566) -> (-7.8372, 13.329)
  line L252 (-7.8372, 13.329) -> (-8.1888, 13.6551)
  line L253 (-8.1888, 13.6551) -> (-8.6246, 13.3099)
  line L254 (-8.6246, 12.8236) -> (-8.6246, 13.2078)
  line L255 (-8.6246, 13.2078) -> (-8.5442, 13.2078)
  line L256 (-8.5442, 13.2078) -> (-8.5442, 13.0648)
  line L257 (-8.5442, 13.0648) -> (-8.0165, 13.0648)
  line L258 (-8.0165, 13.0648) -> (-8.0165, 13.2078)
  line L259 (-8.0165, 13.2078) -> (-7.9444, 13.2078)
  spline S84 degree 2 poles (-7.9444, 13.2078) (-7.9444, 13.1267) (-7.8985, 13.0502) (-7.8347, 13.0451) knots 0 0 0 1 2 2 2
  line L260 (-7.8347, 13.0451) -> (-7.8347, 12.9634)
  line L261 (-7.8347, 12.9634) -> (-8.5442, 12.9634)
  line L262 (-8.5442, 12.9634) -> (-8.5442, 12.8236)
  line L263 (-8.5442, 12.8236) -> (-8.6246, 12.8236)
  line L264 (-8.3541, 12.1722) -> (-8.3541, 12.266)
  line L265 (-8.3541, 12.266) -> (-8.6246, 12.266)
  line L266 (-8.6246, 12.266) -> (-8.6246, 12.3674)
  line L267 (-8.6246, 12.3674) -> (-8.3541, 12.3674)
  line L268 (-8.3541, 12.3674) -> (-8.3541, 12.7152)
  line L269 (-8.3541, 12.7152) -> (-8.2431, 12.7152)
  line L270 (-8.2431, 12.7152) -> (-7.8372, 12.3629)
  line L271 (-7.8372, 12.3629) -> (-7.8372, 12.266)
  line L272 (-7.8372, 12.266) -> (-8.2692, 12.266)
  line L273 (-8.2692, 12.266) -> (-8.2692, 12.1722)
  line L274 (-8.2692, 12.1722) -> (-8.3541, 12.1722)
  line L275 (-8.2692, 12.3674) -> (-7.9617, 12.3674)
  line L276 (-7.9617, 12.3674) -> (-8.2692, 12.6322)
  line L277 (-8.2692, 12.6322) -> (-8.2692, 12.3674)
  spline S85 degree 2 poles (-8.6387, 6.5841) (-8.6387, 6.6696) (-8.6029, 6.7896) (-8.5774, 6.8426) knots 0 0 0 1 2 2 2
  line L278 (-8.5774, 6.8426) -> (-8.446, 6.8426)
  line L279 (-8.446, 6.8426) -> (-8.446, 6.8349)
  spline S86 degree 2 poles (-8.446, 6.8349) (-8.4945, 6.7832) (-8.5481, 6.6524) (-8.5481, 6.5918) knots 0 0 0 1 2 2 2
  spline S87 degree 2 poles (-8.5481, 6.5918) (-8.5481, 6.505) (-8.476, 6.4163) (-8.4166, 6.4163) knots 0 0 0 1 2 2 2
  spline S88 degree 2 poles (-8.4166, 6.4163) (-8.3694, 6.4163) (-8.3107, 6.4629) (-8.296, 6.5133) knots 0 0 0 1 2 2 2
  spline S89 degree 2 poles (-8.296, 6.5133) (-8.2858, 6.5497) (-8.2718, 6.6103) (-8.2603, 6.6556) knots 0 0 0 1 2 2 2
  spline S90 degree 2 poles (-8.2603, 6.6556) (-8.2494, 6.6964) (-8.2169, 6.7609) (-8.1907, 6.7858) knots 0 0 0 1 2 2 2
  spline S91 degree 2 poles (-8.1907, 6.7858) (-8.1646, 6.81) (-8.0944, 6.8368) (-8.0484, 6.8368) knots 0 0 0 1 2 2 2
  spline S92 degree 2 poles (-8.0484, 6.8368) (-7.9527, 6.8368) (-7.8232, 6.6875) (-7.8232, 6.572) knots 0 0 0 1 2 2 2
  spline S93 degree 2 poles (-7.8232, 6.572) (-7.8232, 6.5057) (-7.8494, 6.3882) (-7.8742, 6.3378) knots 0 0 0 1 2 2 2
  line L280 (-7.8742, 6.3378) -> (-7.9993, 6.3378)
  line L281 (-7.9993, 6.3378) -> (-7.9993, 6.3455)
  spline S94 degree 2 poles (-7.9993, 6.3455) (-7.9649, 6.3831) (-7.9138, 6.5005) (-7.9138, 6.565) knots 0 0 0 1 2 2 2
  spline S95 degree 2 poles (-7.9138, 6.565) (-7.9138, 6.6377) (-7.9821, 6.7277) (-8.0376, 6.7277) knots 0 0 0 1 2 2 2
  spline S96 degree 2 poles (-8.0376, 6.7277) (-8.0874, 6.7277) (-8.1467, 6.6747) (-8.1601, 6.625) knots 0 0 0 1 2 2 2
  spline S97 degree 2 poles (-8.1601, 6.625) (-8.169, 6.5918) (-8.192, 6.4954) (-8.2016, 6.4635) knots 0 0 0 1 2 2 2
  spline S98 degree 2 poles (-8.2016, 6.4635) (-8.2265, 6.3825) (-8.3267, 6.3072) (-8.4, 6.3072) knots 0 0 0 1 2 2 2
  spline S99 degree 2 poles (-8.4, 6.3072) (-8.4466, 6.3072) (-8.5359, 6.3449) (-8.5672, 6.3787) knots 0 0 0 1 2 2 2
  spline S100 degree 2 poles (-8.5672, 6.3787) (-8.6017, 6.4163) (-8.6387, 6.512) (-8.6387, 6.5841) knots 0 0 0 1 2 2 2
  line L282 (-8.6246, 5.6264) -> (-8.6246, 5.7623)
  line L283 (-8.6246, 5.7623) -> (-8.2584, 6.0501)
  line L284 (-8.2584, 6.0501) -> (-8.3101, 6.096)
  line L285 (-8.3101, 6.096) -> (-8.6246, 6.096)
  line L286 (-8.6246, 6.096) -> (-8.6246, 6.2006)
  line L287 (-8.6246, 6.2006) -> (-7.8372, 6.2006)
  line L288 (-7.8372, 6.2006) -> (-7.8372, 6.096)
  line L289 (-7.8372, 6.096) -> (-8.199, 6.096)
  line L290 (-8.199, 6.096) -> (-7.8372, 5.7731)
  line L291 (-7.8372, 5.7731) -> (-7.8372, 5.6455)
  line L292 (-7.8372, 5.6455) -> (-8.1888, 5.9716)
  line L293 (-8.1888, 5.9716) -> (-8.6246, 5.6264)
  line L294 (-8.6246, 5.1401) -> (-8.6246, 5.5243)
  line L295 (-8.6246, 5.5243) -> (-8.5442, 5.5243)
  line L296 (-8.5442, 5.5243) -> (-8.5442, 5.3813)
  line L297 (-8.5442, 5.3813) -> (-8.0165, 5.3813)
  line L298 (-8.0165, 5.3813) -> (-8.0165, 5.5243)
  line L299 (-8.0165, 5.5243) -> (-7.9444, 5.5243)
  spline S101 degree 2 poles (-7.9444, 5.5243) (-7.9444, 5.4432) (-7.8985, 5.3667) (-7.8347, 5.3616) knots 0 0 0 1 2 2 2
  line L300 (-7.8347, 5.3616) -> (-7.8347, 5.2799)
  line L301 (-7.8347, 5.2799) -> (-8.5442, 5.2799)
  line L302 (-8.5442, 5.2799) -> (-8.5442, 5.1401)
  line L303 (-8.5442, 5.1401) -> (-8.6246, 5.1401)
  line L304 (-8.3541, 4.4887) -> (-8.3541, 4.5825)
  line L305 (-8.3541, 4.5825) -> (-8.6246, 4.5825)
  line L306 (-8.6246, 4.5825) -> (-8.6246, 4.6839)
  line L307 (-8.6246, 4.6839) -> (-8.3541, 4.6839)
  line L308 (-8.3541, 4.6839) -> (-8.3541, 5.0317)
  line L309 (-8.3541, 5.0317) -> (-8.2431, 5.0317)
  line L310 (-8.2431, 5.0317) -> (-7.8372, 4.6794)
  line L311 (-7.8372, 4.6794) -> (-7.8372, 4.5825)
  line L312 (-7.8372, 4.5825) -> (-8.2692, 4.5825)
  line L313 (-8.2692, 4.5825) -> (-8.2692, 4.4887)
  line L314 (-8.2692, 4.4887) -> (-8.3541, 4.4887)
  line L315 (-8.2692, 4.6839) -> (-7.9617, 4.6839)
  line L316 (-7.9617, 4.6839) -> (-8.2692, 4.9487)
  line L317 (-8.2692, 4.9487) -> (-8.2692, 4.6839)
  spline S102 degree 2 poles (-3.6857, 6.5841) (-3.6857, 6.6696) (-3.6499, 6.7896) (-3.6244, 6.8426) knots 0 0 0 1 2 2 2
  line L318 (-3.6244, 6.8426) -> (-3.493, 6.8426)
  line L319 (-3.493, 6.8426) -> (-3.493, 6.8349)
  spline S103 degree 2 poles (-3.493, 6.8349) (-3.5415, 6.7832) (-3.5951, 6.6524) (-3.5951, 6.5918) knots 0 0 0 1 2 2 2
  spline S104 degree 2 poles (-3.5951, 6.5918) (-3.5951, 6.505) (-3.523, 6.4163) (-3.4636, 6.4163) knots 0 0 0 1 2 2 2
  spline S105 degree 2 poles (-3.4636, 6.4163) (-3.4164, 6.4163) (-3.3577, 6.4629) (-3.343, 6.5133) knots 0 0 0 1 2 2 2
  spline S106 degree 2 poles (-3.343, 6.5133) (-3.3328, 6.5497) (-3.3188, 6.6103) (-3.3073, 6.6556) knots 0 0 0 1 2 2 2
  spline S107 degree 2 poles (-3.3073, 6.6556) (-3.2964, 6.6964) (-3.2639, 6.7609) (-3.2377, 6.7858) knots 0 0 0 1 2 2 2
  spline S108 degree 2 poles (-3.2377, 6.7858) (-3.2116, 6.81) (-3.1414, 6.8368) (-3.0954, 6.8368) knots 0 0 0 1 2 2 2
  spline S109 degree 2 poles (-3.0954, 6.8368) (-2.9997, 6.8368) (-2.8702, 6.6875) (-2.8702, 6.572) knots 0 0 0 1 2 2 2
  spline S110 degree 2 poles (-2.8702, 6.572) (-2.8702, 6.5057) (-2.8964, 6.3882) (-2.9212, 6.3378) knots 0 0 0 1 2 2 2
  line L320 (-2.9212, 6.3378) -> (-3.0463, 6.3378)
  line L321 (-3.0463, 6.3378) -> (-3.0463, 6.3455)
  spline S111 degree 2 poles (-3.0463, 6.3455) (-3.0119, 6.3831) (-2.9608, 6.5005) (-2.9608, 6.565) knots 0 0 0 1 2 2 2
  spline S112 degree 2 poles (-2.9608, 6.565) (-2.9608, 6.6377) (-3.0291, 6.7277) (-3.0846, 6.7277) knots 0 0 0 1 2 2 2
  spline S113 degree 2 poles (-3.0846, 6.7277) (-3.1344, 6.7277) (-3.1937, 6.6747) (-3.2071, 6.625) knots 0 0 0 1 2 2 2
  spline S114 degree 2 poles (-3.2071, 6.625) (-3.216, 6.5918) (-3.239, 6.4954) (-3.2486, 6.4635) knots 0 0 0 1 2 2 2
  spline S115 degree 2 poles (-3.2486, 6.4635) (-3.2735, 6.3825) (-3.3737, 6.3072) (-3.447, 6.3072) knots 0 0 0 1 2 2 2
  spline S116 degree 2 poles (-3.447, 6.3072) (-3.4936, 6.3072) (-3.5829, 6.3449) (-3.6142, 6.3787) knots 0 0 0 1 2 2 2
  spline S117 degree 2 poles (-3.6142, 6.3787) (-3.6487, 6.4163) (-3.6857, 6.512) (-3.6857, 6.5841) knots 0 0 0 1 2 2 2
  line L322 (-3.6716, 5.6264) -> (-3.6716, 5.7623)
  line L323 (-3.6716, 5.7623) -> (-3.3054, 6.0501)
  line L324 (-3.3054, 6.0501) -> (-3.3571, 6.096)
  line L325 (-3.3571, 6.096) -> (-3.6716, 6.096)
  line L326 (-3.6716, 6.096) -> (-3.6716, 6.2006)
  line L327 (-3.6716, 6.2006) -> (-2.8842, 6.2006)
  line L328 (-2.8842, 6.2006) -> (-2.8842, 6.096)
  line L329 (-2.8842, 6.096) -> (-3.246, 6.096)
  line L330 (-3.246, 6.096) -> (-2.8842, 5.7731)
  line L331 (-2.8842, 5.7731) -> (-2.8842, 5.6455)
  line L332 (-2.8842, 5.6455) -> (-3.2358, 5.9716)
  line L333 (-3.2358, 5.9716) -> (-3.6716, 5.6264)
  line L334 (-3.6716, 5.1401) -> (-3.6716, 5.5243)
  line L335 (-3.6716, 5.5243) -> (-3.5912, 5.5243)
  line L336 (-3.5912, 5.5243) -> (-3.5912, 5.3813)
  line L337 (-3.5912, 5.3813) -> (-3.0635, 5.3813)
  line L338 (-3.0635, 5.3813) -> (-3.0635, 5.5243)
  line L339 (-3.0635, 5.5243) -> (-2.9914, 5.5243)
  spline S118 degree 2 poles (-2.9914, 5.5243) (-2.9914, 5.4432) (-2.9455, 5.3667) (-2.8817, 5.3616) knots 0 0 0 1 2 2 2
  line L340 (-2.8817, 5.3616) -> (-2.8817, 5.2799)
  line L341 (-2.8817, 5.2799) -> (-3.5912, 5.2799)
  line L342 (-3.5912, 5.2799) -> (-3.5912, 5.1401)
  line L343 (-3.5912, 5.1401) -> (-3.6716, 5.1401)
  line L344 (-3.4011, 4.4887) -> (-3.4011, 4.5825)
  line L345 (-3.4011, 4.5825) -> (-3.6716, 4.5825)
  line L346 (-3.6716, 4.5825) -> (-3.6716, 4.6839)
  line L347 (-3.6716, 4.6839) -> (-3.4011, 4.6839)
  line L348 (-3.4011, 4.6839) -> (-3.4011, 5.0317)
  line L349 (-3.4011, 5.0317) -> (-3.2901, 5.0317)
  line L350 (-3.2901, 5.0317) -> (-2.8842, 4.6794)
  line L351 (-2.8842, 4.6794) -> (-2.8842, 4.5825)
  line L352 (-2.8842, 4.5825) -> (-3.3162, 4.5825)
  line L353 (-3.3162, 4.5825) -> (-3.3162, 4.4887)
  line L354 (-3.3162, 4.4887) -> (-3.4011, 4.4887)
  line L355 (-3.3162, 4.6839) -> (-3.0087, 4.6839)
  line L356 (-3.0087, 4.6839) -> (-3.3162, 4.9487)
  line L357 (-3.3162, 4.9487) -> (-3.3162, 4.6839)
  spline S119 degree 2 poles (-3.6857, 14.2676) (-3.6857, 14.3531) (-3.6499, 14.4731) (-3.6244, 14.5261) knots 0 0 0 1 2 2 2
  line L358 (-3.6244, 14.5261) -> (-3.493, 14.5261)
  line L359 (-3.493, 14.5261) -> (-3.493, 14.5184)
  spline S120 degree 2 poles (-3.493, 14.5184) (-3.5415, 14.4667) (-3.5951, 14.3359) (-3.5951, 14.2753) knots 0 0 0 1 2 2 2
  spline S121 degree 2 poles (-3.5951, 14.2753) (-3.5951, 14.1885) (-3.523, 14.0998) (-3.4636, 14.0998) knots 0 0 0 1 2 2 2
  spline S122 degree 2 poles (-3.4636, 14.0998) (-3.4164, 14.0998) (-3.3577, 14.1464) (-3.343, 14.1968) knots 0 0 0 1 2 2 2
  spline S123 degree 2 poles (-3.343, 14.1968) (-3.3328, 14.2332) (-3.3188, 14.2938) (-3.3073, 14.3391) knots 0 0 0 1 2 2 2
  spline S124 degree 2 poles (-3.3073, 14.3391) (-3.2964, 14.3799) (-3.2639, 14.4444) (-3.2377, 14.4693) knots 0 0 0 1 2 2 2
  spline S125 degree 2 poles (-3.2377, 14.4693) (-3.2116, 14.4935) (-3.1414, 14.5203) (-3.0954, 14.5203) knots 0 0 0 1 2 2 2
  spline S126 degree 2 poles (-3.0954, 14.5203) (-2.9997, 14.5203) (-2.8702, 14.371) (-2.8702, 14.2555) knots 0 0 0 1 2 2 2
  spline S127 degree 2 poles (-2.8702, 14.2555) (-2.8702, 14.1892) (-2.8964, 14.0717) (-2.9212, 14.0213) knots 0 0 0 1 2 2 2
  line L360 (-2.9212, 14.0213) -> (-3.0463, 14.0213)
  line L361 (-3.0463, 14.0213) -> (-3.0463, 14.029)
  spline S128 degree 2 poles (-3.0463, 14.029) (-3.0119, 14.0666) (-2.9608, 14.184) (-2.9608, 14.2485) knots 0 0 0 1 2 2 2
  spline S129 degree 2 poles (-2.9608, 14.2485) (-2.9608, 14.3212) (-3.0291, 14.4112) (-3.0846, 14.4112) knots 0 0 0 1 2 2 2
  spline S130 degree 2 poles (-3.0846, 14.4112) (-3.1344, 14.4112) (-3.1937, 14.3582) (-3.2071, 14.3085) knots 0 0 0 1 2 2 2
  spline S131 degree 2 poles (-3.2071, 14.3085) (-3.216, 14.2753) (-3.239, 14.1789) (-3.2486, 14.147) knots 0 0 0 1 2 2 2
  spline S132 degree 2 poles (-3.2486, 14.147) (-3.2735, 14.066) (-3.3737, 13.9907) (-3.447, 13.9907) knots 0 0 0 1 2 2 2
  spline S133 degree 2 poles (-3.447, 13.9907) (-3.4936, 13.9907) (-3.5829, 14.0284) (-3.6142, 14.0622) knots 0 0 0 1 2 2 2
  spline S134 degree 2 poles (-3.6142, 14.0622) (-3.6487, 14.0998) (-3.6857, 14.1955) (-3.6857, 14.2676) knots 0 0 0 1 2 2 2
  line L362 (-3.6716, 13.3099) -> (-3.6716, 13.4458)
  line L363 (-3.6716, 13.4458) -> (-3.3054, 13.7336)
  line L364 (-3.3054, 13.7336) -> (-3.3571, 13.7795)
  line L365 (-3.3571, 13.7795) -> (-3.6716, 13.7795)
  line L366 (-3.6716, 13.7795) -> (-3.6716, 13.8841)
  line L367 (-3.6716, 13.8841) -> (-2.8842, 13.8841)
  line L368 (-2.8842, 13.8841) -> (-2.8842, 13.7795)
  line L369 (-2.8842, 13.7795) -> (-3.246, 13.7795)
  line L370 (-3.246, 13.7795) -> (-2.8842, 13.4566)
  line L371 (-2.8842, 13.4566) -> (-2.8842, 13.329)
  line L372 (-2.8842, 13.329) -> (-3.2358, 13.6551)
  line L373 (-3.2358, 13.6551) -> (-3.6716, 13.3099)
  line L374 (-3.6716, 12.8236) -> (-3.6716, 13.2078)
  line L375 (-3.6716, 13.2078) -> (-3.5912, 13.2078)
  line L376 (-3.5912, 13.2078) -> (-3.5912, 13.0648)
  line L377 (-3.5912, 13.0648) -> (-3.0635, 13.0648)
  line L378 (-3.0635, 13.0648) -> (-3.0635, 13.2078)
  line L379 (-3.0635, 13.2078) -> (-2.9914, 13.2078)
  spline S135 degree 2 poles (-2.9914, 13.2078) (-2.9914, 13.1267) (-2.9455, 13.0502) (-2.8817, 13.0451) knots 0 0 0 1 2 2 2
  line L380 (-2.8817, 13.0451) -> (-2.8817, 12.9634)
  line L381 (-2.8817, 12.9634) -> (-3.5912, 12.9634)
  line L382 (-3.5912, 12.9634) -> (-3.5912, 12.8236)
  line L383 (-3.5912, 12.8236) -> (-3.6716, 12.8236)
  line L384 (-3.4011, 12.1722) -> (-3.4011, 12.266)
  line L385 (-3.4011, 12.266) -> (-3.6716, 12.266)
  line L386 (-3.6716, 12.266) -> (-3.6716, 12.3674)
  line L387 (-3.6716, 12.3674) -> (-3.4011, 12.3674)
  line L388 (-3.4011, 12.3674) -> (-3.4011, 12.7152)
  line L389 (-3.4011, 12.7152) -> (-3.2901, 12.7152)
  line L390 (-3.2901, 12.7152) -> (-2.8842, 12.3629)
  line L391 (-2.8842, 12.3629) -> (-2.8842, 12.266)
  line L392 (-2.8842, 12.266) -> (-3.3162, 12.266)
  line L393 (-3.3162, 12.266) -> (-3.3162, 12.1722)
  line L394 (-3.3162, 12.1722) -> (-3.4011, 12.1722)
  line L395 (-3.3162, 12.3674) -> (-3.0087, 12.3674)
  line L396 (-3.0087, 12.3674) -> (-3.3162, 12.6322)
  line L397 (-3.3162, 12.6322) -> (-3.3162, 12.3674)
  spline S136 degree 2 poles (1.2673, 14.2676) (1.2673, 14.3531) (1.3031, 14.4731) (1.3286, 14.5261) knots 0 0 0 1 2 2 2
  line L398 (1.3286, 14.5261) -> (1.46, 14.5261)
  line L399 (1.46, 14.5261) -> (1.46, 14.5184)
  spline S137 degree 2 poles (1.46, 14.5184) (1.4115, 14.4667) (1.3579, 14.3359) (1.3579, 14.2753) knots 0 0 0 1 2 2 2
  spline S138 degree 2 poles (1.3579, 14.2753) (1.3579, 14.1885) (1.43, 14.0998) (1.4894, 14.0998) knots 0 0 0 1 2 2 2
  spline S139 degree 2 poles (1.4894, 14.0998) (1.5366, 14.0998) (1.5953, 14.1464) (1.61, 14.1968) knots 0 0 0 1 2 2 2
  spline S140 degree 2 poles (1.61, 14.1968) (1.6202, 14.2332) (1.6342, 14.2938) (1.6457, 14.3391) knots 0 0 0 1 2 2 2
  spline S141 degree 2 poles (1.6457, 14.3391) (1.6566, 14.3799) (1.6891, 14.4444) (1.7153, 14.4693) knots 0 0 0 1 2 2 2
  spline S142 degree 2 poles (1.7153, 14.4693) (1.7414, 14.4935) (1.8116, 14.5203) (1.8576, 14.5203) knots 0 0 0 1 2 2 2
  spline S143 degree 2 poles (1.8576, 14.5203) (1.9533, 14.5203) (2.0828, 14.371) (2.0828, 14.2555) knots 0 0 0 1 2 2 2
  spline S144 degree 2 poles (2.0828, 14.2555) (2.0828, 14.1892) (2.0566, 14.0717) (2.0318, 14.0213) knots 0 0 0 1 2 2 2
  line L400 (2.0318, 14.0213) -> (1.9067, 14.0213)
  line L401 (1.9067, 14.0213) -> (1.9067, 14.029)
  spline S145 degree 2 poles (1.9067, 14.029) (1.9411, 14.0666) (1.9922, 14.184) (1.9922, 14.2485) knots 0 0 0 1 2 2 2
  spline S146 degree 2 poles (1.9922, 14.2485) (1.9922, 14.3212) (1.9239, 14.4112) (1.8684, 14.4112) knots 0 0 0 1 2 2 2
  spline S147 degree 2 poles (1.8684, 14.4112) (1.8186, 14.4112) (1.7593, 14.3582) (1.7459, 14.3085) knots 0 0 0 1 2 2 2
  spline S148 degree 2 poles (1.7459, 14.3085) (1.737, 14.2753) (1.714, 14.1789) (1.7044, 14.147) knots 0 0 0 1 2 2 2
  spline S149 degree 2 poles (1.7044, 14.147) (1.6795, 14.066) (1.5793, 13.9907) (1.506, 13.9907) knots 0 0 0 1 2 2 2
  spline S150 degree 2 poles (1.506, 13.9907) (1.4594, 13.9907) (1.3701, 14.0284) (1.3388, 14.0622) knots 0 0 0 1 2 2 2
  spline S151 degree 2 poles (1.3388, 14.0622) (1.3043, 14.0998) (1.2673, 14.1955) (1.2673, 14.2676) knots 0 0 0 1 2 2 2
  line L402 (1.2814, 13.3099) -> (1.2814, 13.4458)
  line L403 (1.2814, 13.4458) -> (1.6476, 13.7336)
  line L404 (1.6476, 13.7336) -> (1.5959, 13.7795)
  line L405 (1.5959, 13.7795) -> (1.2814, 13.7795)
  line L406 (1.2814, 13.7795) -> (1.2814, 13.8841)
  line L407 (1.2814, 13.8841) -> (2.0688, 13.8841)
  line L408 (2.0688, 13.8841) -> (2.0688, 13.7795)
  line L409 (2.0688, 13.7795) -> (1.707, 13.7795)
  line L410 (1.707, 13.7795) -> (2.0688, 13.4566)
  line L411 (2.0688, 13.4566) -> (2.0688, 13.329)
  line L412 (2.0688, 13.329) -> (1.7172, 13.6551)
  line L413 (1.7172, 13.6551) -> (1.2814, 13.3099)
  line L414 (1.2814, 12.8236) -> (1.2814, 13.2078)
  line L415 (1.2814, 13.2078) -> (1.3618, 13.2078)
  line L416 (1.3618, 13.2078) -> (1.3618, 13.0648)
  line L417 (1.3618, 13.0648) -> (1.8895, 13.0648)
  line L418 (1.8895, 13.0648) -> (1.8895, 13.2078)
  line L419 (1.8895, 13.2078) -> (1.9616, 13.2078)
  spline S152 degree 2 poles (1.9616, 13.2078) (1.9616, 13.1267) (2.0075, 13.0502) (2.0713, 13.0451) knots 0 0 0 1 2 2 2
  line L420 (2.0713, 13.0451) -> (2.0713, 12.9634)
  line L421 (2.0713, 12.9634) -> (1.3618, 12.9634)
  line L422 (1.3618, 12.9634) -> (1.3618, 12.8236)
  line L423 (1.3618, 12.8236) -> (1.2814, 12.8236)
  line L424 (1.5519, 12.1722) -> (1.5519, 12.266)
  line L425 (1.5519, 12.266) -> (1.2814, 12.266)
  line L426 (1.2814, 12.266) -> (1.2814, 12.3674)
  line L427 (1.2814, 12.3674) -> (1.5519, 12.3674)
  line L428 (1.5519, 12.3674) -> (1.5519, 12.7152)
  line L429 (1.5519, 12.7152) -> (1.6629, 12.7152)
  line L430 (1.6629, 12.7152) -> (2.0688, 12.3629)
  line L431 (2.0688, 12.3629) -> (2.0688, 12.266)
  line L432 (2.0688, 12.266) -> (1.6368, 12.266)
  line L433 (1.6368, 12.266) -> (1.6368, 12.1722)
  line L434 (1.6368, 12.1722) -> (1.5519, 12.1722)
  line L435 (1.6368, 12.3674) -> (1.9443, 12.3674)
  line L436 (1.9443, 12.3674) -> (1.6368, 12.6322)
  line L437 (1.6368, 12.6322) -> (1.6368, 12.3674)
  spline S153 degree 2 poles (1.2673, 6.5841) (1.2673, 6.6696) (1.3031, 6.7896) (1.3286, 6.8426) knots 0 0 0 1 2 2 2
  line L438 (1.3286, 6.8426) -> (1.46, 6.8426)
  line L439 (1.46, 6.8426) -> (1.46, 6.8349)
  spline S154 degree 2 poles (1.46, 6.8349) (1.4115, 6.7832) (1.3579, 6.6524) (1.3579, 6.5918) knots 0 0 0 1 2 2 2
  spline S155 degree 2 poles (1.3579, 6.5918) (1.3579, 6.505) (1.43, 6.4163) (1.4894, 6.4163) knots 0 0 0 1 2 2 2
  spline S156 degree 2 poles (1.4894, 6.4163) (1.5366, 6.4163) (1.5953, 6.4629) (1.61, 6.5133) knots 0 0 0 1 2 2 2
  spline S157 degree 2 poles (1.61, 6.5133) (1.6202, 6.5497) (1.6342, 6.6103) (1.6457, 6.6556) knots 0 0 0 1 2 2 2
  spline S158 degree 2 poles (1.6457, 6.6556) (1.6566, 6.6964) (1.6891, 6.7609) (1.7153, 6.7858) knots 0 0 0 1 2 2 2
  spline S159 degree 2 poles (1.7153, 6.7858) (1.7414, 6.81) (1.8116, 6.8368) (1.8576, 6.8368) knots 0 0 0 1 2 2 2
  spline S160 degree 2 poles (1.8576, 6.8368) (1.9533, 6.8368) (2.0828, 6.6875) (2.0828, 6.572) knots 0 0 0 1 2 2 2
  spline S161 degree 2 poles (2.0828, 6.572) (2.0828, 6.5057) (2.0566, 6.3882) (2.0318, 6.3378) knots 0 0 0 1 2 2 2
  line L440 (2.0318, 6.3378) -> (1.9067, 6.3378)
  line L441 (1.9067, 6.3378) -> (1.9067, 6.3455)
  spline S162 degree 2 poles (1.9067, 6.3455) (1.9411, 6.3831) (1.9922, 6.5005) (1.9922, 6.565) knots 0 0 0 1 2 2 2
  spline S163 degree 2 poles (1.9922, 6.565) (1.9922, 6.6377) (1.9239, 6.7277) (1.8684, 6.7277) knots 0 0 0 1 2 2 2
  spline S164 degree 2 poles (1.8684, 6.7277) (1.8186, 6.7277) (1.7593, 6.6747) (1.7459, 6.625) knots 0 0 0 1 2 2 2
  spline S165 degree 2 poles (1.7459, 6.625) (1.737, 6.5918) (1.714, 6.4954) (1.7044, 6.4635) knots 0 0 0 1 2 2 2
  spline S166 degree 2 poles (1.7044, 6.4635) (1.6795, 6.3825) (1.5793, 6.3072) (1.506, 6.3072) knots 0 0 0 1 2 2 2
  spline S167 degree 2 poles (1.506, 6.3072) (1.4594, 6.3072) (1.3701, 6.3449) (1.3388, 6.3787) knots 0 0 0 1 2 2 2
  spline S168 degree 2 poles (1.3388, 6.3787) (1.3043, 6.4163) (1.2673, 6.512) (1.2673, 6.5841) knots 0 0 0 1 2 2 2
  line L442 (1.2814, 5.6264) -> (1.2814, 5.7623)
  line L443 (1.2814, 5.7623) -> (1.6476, 6.0501)
  line L444 (1.6476, 6.0501) -> (1.5959, 6.096)
  line L445 (1.5959, 6.096) -> (1.2814, 6.096)
  line L446 (1.2814, 6.096) -> (1.2814, 6.2006)
  line L447 (1.2814, 6.2006) -> (2.0688, 6.2006)
  line L448 (2.0688, 6.2006) -> (2.0688, 6.096)
  line L449 (2.0688, 6.096) -> (1.707, 6.096)
  line L450 (1.707, 6.096) -> (2.0688, 5.7731)
  line L451 (2.0688, 5.7731) -> (2.0688, 5.6455)